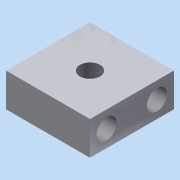
# Autodesk Inventor part: Extruder mount top
Saved by Autodesk Inventor 2015 (Build 190159000, 159)
## iProperties
Created: 2016-06-25
Part Number: Extruder mount top
Material: Generic
Document SubType Name: Modeling
Designer: Dustin
Density: 1 g/cm^3
Appearance: Default
Author: Dustin
Autodesk Inventor part; units mm, degrees
ref_plane "YZ Plane" through (0, 0, 0) normal (1, 0, 0) x (0, 1, 0)
ref_plane "XZ Plane" through (0, 0, 0) normal (0, 1, 0) x (-1, 0, 0)
ref_plane "XY Plane" through (0, 0, 0) normal (0, 0, 1) x (1, 0, 0)
sketch "Sketch1" plane through (0, 0, 0) normal (0, 1, 0) x (-1, 0, 0)
  line L0 (0, 0) -> (50, 0)
  line L1 (50, 0) -> (50, -50)
  line L2 (50, -50) -> (0, -50)
  line L3 (0, -50) -> (0, 0)
  dimension "d0" = 50
  dimension "d1" = 50
  constraints: 8 end point, 2 parallel, 1 horizontal, 1 perpendicular
  measures "d0" distance of L0.start L0.end
  measures "d1" distance of L2.end L0.start
extrude "Extrusion1" add sketch "Sketch1" along normal blind 20
sketch "Sketch2" plane through (0, 0, 0) normal (1, 0, 0) x (0, 0, -1)
  line L0 (0, 20) -> (50, 20) projected
  line L1 (0, 0) -> (0, 20) projected
  line L2 (50, 0) -> (50, 20) projected
  point P0 (10, 10)
  point P1 (40, 10)
  dimension "d4" = 10
  dimension "d5" = 10
  dimension "d6" = 10
  dimension "d7" = 10
  measures "d4" distance from line of L0 point (10, 10)
  measures "d5" distance from line of L0 point (40, 10)
  measures "d6" distance from line of L1 point (10, 10)
  measures "d7" distance from line of L2 point (40, 10)
hole "Hole1" at (0, 10, -10) at (0, 10, -40) direction (-1, 0, 0) diameter 12 depth 50 tip angle 118
sketch "Sketch3" plane through (0, 20, 0) normal (0, 1, 0) x (1, 0, 0)
  line L0 (-50, 0) -> (-50, 50) projected
  line L1 (0, 50) -> (-50, 50) projected
  point P0 (0, 0)
  point P1 (-25, 25)
  dimension "d15" = 25
  dimension "d16" = 25
  measures "d15" distance from line of L0 point (-25, 25)
  measures "d16" distance from line of L1 point (-25, 25)
hole "Hole2" at (-25, 20, -25) direction (0, -1, 0) diameter 12 depth 50 tip angle 118
body "Solid1"
